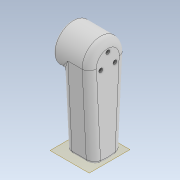
# Autodesk Inventor part: shank_link
Saved by Autodesk Inventor 2020 (Build 240168000, 168)
## iProperties
Created: 2020-12-22
Part Number: shank_link
Material: Generic
Document SubType Name: Modeling
Designer: DELL
Density: 1 g/cm^3
Appearance: Default
Author: DELL
Autodesk Inventor part; units mm, degrees
ref_plane "XY Plane" through (0, 0, 0) normal (0, 0, 1) x (1, 0, 0)
sketch "Sketch1" plane through (0, 0, 0) normal (1, 0, 0) x (0, 1, 0)
  line L0 (0, 0) -> (0, 25.2399) construction
  line L1 (0, 0) -> (0, -46.7601) construction
  line L2 (0, 0) -> (-120, 0) construction
  circle A0 centre (0, 0) radius 26
  line L3 (0, 0) -> (-13, 22.5167) construction
  line L4 (0, 0) -> (-13, -22.5167) construction
  line L5 (-1.3055, 25.9672) -> (-120, 20)
  line L6 (-1.3055, -25.9672) -> (-120, -20)
  line L7 (-120, 20) -> (-120, -20)
  circle A1 centre (0, 0) radius 11.5 construction
  circle A2 centre (11.5, 0) radius 1.65
  line L8 (0, 0) -> (26, 0) construction
  circle A3 centre (-5.75, 9.9593) radius 1.65
  circle A4 centre (-5.75, -9.9593) radius 1.65
  circle A5 centre (0, 0) radius 9.715 construction
  line L9 (0, 0) -> (5.75, 9.9593) construction
  line L10 (0, 0) -> (5.75, -9.9593) construction
  circle A6 centre (4.8575, 8.4134) radius 2
  circle A7 centre (4.8575, -8.4134) radius 2
  circle A8 centre (-9.715, 0) radius 2
  circle A9 centre (11.5, 0) radius 2.75
  circle A10 centre (-5.75, -9.9593) radius 2.75
  circle A11 centre (-5.75, 9.9593) radius 2.75
  circle A12 centre (-60, 0) radius 60 construction
  arc A13 (-116.5061, 20.1756) -> (-116.5061, -20.1756) centre (-60, 0) ccw
  point P0 (-60, 0)
  point P1 (20.1084, 33.9985)
  dimension "d6" = 52
  dimension "d8" = 60
  dimension "d84" = 120
  dimension "d85" = 40
  dimension "d97" = 23
  dimension "d98" = 3.3
  dimension "d99" = 19.43
  dimension "d100" = 30
  dimension "d101" = 4
  dimension "d102" = 5.5
  dimension "d122" = 120
  constraints: 22 end point, 18 point on circle, 14 centre point, 9 point on line, 7 coincident, 6 equal radius, 3 midpoint, 2 vertical, 1 horizontal, 1 perpendicular, 1 symmetric about line, 1 tangent, 3 other
  measures "d6" diameter of A0
  measures "d8" angle of L2 L3
  measures "d84" distance between parallel lines of L7 L1
  measures "d85" distance of L5.end L6.end
  measures "d97" diameter of A1
  measures "d98" diameter of A2
  measures "d99" diameter of A5
  measures "d100" angle of L0 L9
  measures "d101" diameter of A6
  measures "d102" diameter of A9
  measures "d122" diameter of A12
ref_plane "Work Plane1" through (14.5, 0, 0) normal (1, 0, 0) x (0, 1, 0)
ref_plane "Work Plane2" through (-14.5, 0, 0) normal (1, 0, 0) x (0, 1, 0)
extrude "Extrusion1" [suppressed]
extrude "Extrusion2" [suppressed]
extrude "Extrusion4" add sketch "Sketch1" along normal blind 20 and the other way blind 30 contours A0 | A6 | A7 | A8 | A9 | A10 | A11
extrude "Extrusion6" cut sketch "Sketch1" against normal blind 40 from surface at 20 contours A9 | A10 | A11
extrude "Extrusion7" cut sketch "Sketch1" along normal blind 5 from surface at -30 contours A6 | A7 | A8
extrude "Extrusion9" add sketch "Sketch1" along normal mid plane 40 contours A0 L6 A13 L5
sketch "Sketch6" plane through (0, 0, 0) normal (0, 1, 0) x (-1, 0, 0)
  circle A0 centre (0, 0) radius 10
  dimension "d123" = 20
  constraints: 1 centre point, 1 coincident
  measures "d123" diameter of A0
ref_plane "Work Plane4" through (0, -120, 0) normal (0, 1, 0) x (-1, 0, 0)
extrude "Extrusion11" cut sketch "Sketch6" along normal blind 60 from surface at -120
fillet "Fillet28" radius 10 4 edges at (20, -58.9058, 23.0714) (-20, -58.9058, 23.0714) (20, -58.9058, -23.0714) (-20, -58.9058, -23.0714)
fillet "Fillet29" radius 4 8 edges at (16.5726, -117.3399, 17.6673) (20, -120, 0) (16.5726, -117.3399, -17.6672) (0, -116.5061, -20.1756) (-16.5579, -117.3359, -17.6803) (-20, -120, 0) (-16.5726, -117.3399, 17.6673) (0, -116.5061, 20.1756)
fillet "Fillet31" radius 2 1 edges at (-30, -26, 0)
fillet "Fillet32" radius 5 3 edges at (-20, -26, 0) (-16.2427, -11.622, -23.2579) (-16.2439, -11.6241, 23.2568)
fillet "Fillet33" radius 2 3 edges at (-0.0119, -119.1608, 10) (-0.0113, -119.1608, -10) (10, -60, 0)
body "Solid1"
